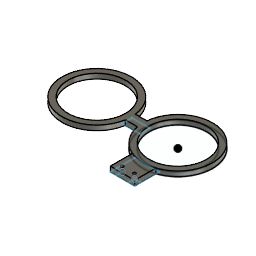
dual_holder_minicups_i1 (Autodesk Fusion 360 design; units mm, degrees)
part number: 2026-05-12-01-25-46-114
Autodesk Fusion 360 part; units mm, degrees
sketch "Sketch1" plane through (0, 0, 0) normal (0, 0, 1) x (1, 0, 0)
  circle A0 centre (0, 0) radius 29
  circle A1 centre (0, 0) radius 35
  line L0 (-13.6747, -29.8699) -> (11.0253, -29.8699)
  line L1 (11.0253, -29.8699) -> (11.0253, -54.5699)
  line L2 (11.0253, -54.5699) -> (-13.6747, -54.5699)
  line L3 (-13.6747, -54.5699) -> (-13.6747, -29.8699)
  line L4 (-31.8811, 3.5534) -> (-49.8811, 3.5534)
  line L5 (-49.8811, 3.5534) -> (-49.8811, -6.4466)
  line L6 (-49.8811, -6.4466) -> (-31.8811, -6.4466)
  line L7 (-31.8811, -6.4466) -> (-31.8811, 3.5534)
  line L8 (-13.6747, -48.6199) -> (-7.4997, -48.6199)
  line L9 (-7.4997, -54.5699) -> (-7.4997, -48.6199)
  line L10 (11.0253, -48.6199) -> (4.8503, -48.6199)
  line L11 (4.8719, -54.5699) -> (4.8719, -48.6199)
  circle A2 centre (4.8503, -48.6199) radius 1.3
  circle A3 centre (-7.4997, -48.6199) radius 1.3
  dimension "d3" = 58
  dimension "d4" = 70
  dimension "d12" = 24.7
  dimension "d13" = 24.7
  dimension "d14" = 18
  dimension "d15" = 10
  dimension "d18" = 6.175
  dimension "d19" = 5.95
  dimension "d20" = 6.175
  dimension "d21" = 5.95
  dimension "d23" = 2.6
  dimension "d24" = 2.6
  constraint coincident A0.centre A1.centre
  constraint concentric A0 A1
  constraint horizontal L0
  constraint vertical L1
  constraint horizontal L2
  constraint vertical L3
  constraint horizontal L4
  constraint vertical L5
  constraint horizontal L6
  constraint vertical L7
  constraint coincident L3 L8.start
  constraint perpendicular L3 L8
  constraint coincident L2 L9.start
  constraint perpendicular L2 L9
  constraint coincident L1 L10.start
  constraint perpendicular L1 L10
  constraint coincident L2 L11.start
  constraint perpendicular L10 L11
  constraint coincident L10.end A2.centre
  constraint coincident L8.end L9.end
  measures "d3" diameter of A0
  measures "d4" diameter of A1
  measures "d12" distance of L0.start L0.end
  measures "d13" distance of L0.start L2.end
  measures "d14" distance of L4.start L4.end
  measures "d15" distance of L4.start L6.end
  measures "d18" distance of L8.start L8.end
  measures "d19" distance of L8.end L9.start
  measures "d20" distance of L10.start L10.end
  measures "d21" distance of L11.start L11.end
  measures "d23" diameter of A2
  measures "d24" diameter of A3
extrude "Extrude1" add sketch "Sketch1" along normal blind 5 contours A1 L0 L1 L3 L4 L6 L7 | A1 L4 L6 L7 | A1 L0 L1 L3 makes body 1
extrude "Extrude2" add sketch "Sketch1" along normal blind 5 separate body contours A1 L1 L2 L3 L8 L9 L10 L11 A2 A3 | L1 L2 L10 L11 A2 | L2 L3 L8 L9 A3 makes body 2
sketch "Sketch2" plane through (0, 0, 0) normal (0, 0, 1) x (1, 0, 0)
  circle A0 centre (-81.102, -0.73) radius 29
  circle A1 centre (-81.102, -0.73) radius 35
  dimension "d27" = 58
  dimension "d28" = 70
  constraint concentric A0 A1
  measures "d27" diameter of A0
  measures "d28" diameter of A1
extrude "Extrude3" add sketch "Sketch1" sketch "Sketch2" along normal blind 5 contours A1 L4 L5 L6 of sketch 2 bodies 1
equation "holder_d = 58 mm"
equation "holder_od = holder_d + 12 mm"
equation "d3 = holder_d"
equation "d4 = holder_od"
equation "d5 = holder_thickness"
equation "holder_thickness = 5 mm"
equation "mount_w = 24.7 mm"
equation "mount_l = 24.7 mm"
equation "connecter_w = 10 mm"
equation "connecter_l = 18 mm"
equation "d12 = mount_w"
equation "d13 = mount_l"
equation "d14 = connecter_l"
equation "d15 = connecter_w"
equation "offset_m3hole_w = 6.175 mm"
equation "offset_m3hole_l = 5.95 mm"
equation "d18 = offset_m3hole_w"
equation "d19 = offset_m3hole_l"
equation "d20 = offset_m3hole_w"
equation "m3_diam = 2.6 mm"
equation "d23 = m3_diam"
equation "d24 = m3_diam"
equation "d25 = holder_thickness"
equation "d27 = holder_d"
equation "d28 = holder_od"
equation "d29 = holder_thickness"
